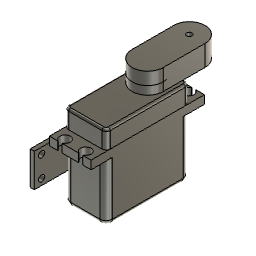
Servo v3 (Autodesk Fusion 360 design; units mm, degrees)
Autodesk Fusion 360 part; units mm, degrees
note: some values were not read from the file. Set by a fixed rule: which sketch regions a step uses.
sketch "Sketch1" plane through (0, 0, 0) normal (0, 0, 1) x (1, 0, 0)
  line L0 (0, 0) -> (20, 0)
  line L1 (20, 0) -> (20, 40)
  line L2 (20, 40) -> (0, 40)
  line L3 (0, 40) -> (0, 0)
  dimension "d1" = 20
  dimension "d2" = 40
  constraint horizontal L0
  constraint vertical L1
  constraint horizontal L2
  constraint vertical L3
  constraint coincident L0.start L3.end
  measures "d1" distance of L1.end L2.end
  measures "d2" distance of L0.end L1.end
extrude "Extrude1" add sketch "Sketch1" along normal blind 27.7 makes body 1
sketch "Sketch2" plane through (0, 0, 27.7) normal (0, 0, 1) x (-1, 0, 0)
  line L0 (0, -40) -> (0, 0)
  line L1 (0, 0) -> (-20, 0)
  line L2 (-20, 0) -> (-20, -40)
  line L3 (-20, -40) -> (0, -40)
  line L4 (0, -47.25) -> (-20, -47.25)
  line L5 (-20, -47.25) -> (-20, 7.25)
  line L6 (-20, 7.25) -> (0, 7.25)
  line L7 (0, 7.25) -> (0, -47.25)
  circle A0 centre (-5, -44.75) radius 2.5
  circle A1 centre (-15, -44.75) radius 2.5
  circle A2 centre (-15, 4.75) radius 2.5
  circle A3 centre (-5, 4.75) radius 2.5
  line L8 (-10, -47.25) -> (-10, 7.25)
  line L9 (-4, -47.25) -> (-6, -47.25)
  line L10 (-6, -47.25) -> (-6, -46.3307)
  line L11 (-6, -46.3307) -> (-4, -46.3307)
  line L12 (-4, -46.3307) -> (-4, -47.25)
  line L13 (-14, -47.25) -> (-16, -47.25)
  line L14 (-16, -47.25) -> (-16, -46.3307)
  line L15 (-16, -46.3307) -> (-14, -46.3307)
  line L16 (-14, -46.3307) -> (-14, -47.25)
  line L17 (-14, 6.8523) -> (-16, 6.8523)
  line L18 (-16, 6.8523) -> (-16, 7.25)
  line L19 (-16, 7.25) -> (-14, 7.25)
  line L20 (-14, 7.25) -> (-14, 6.8523)
  line L21 (-4, 6.8576) -> (-6, 6.8576)
  line L22 (-6, 6.8576) -> (-6, 7.25)
  line L23 (-6, 7.25) -> (-4, 7.25)
  line L24 (-4, 7.25) -> (-4, 6.8576)
  dimension "d5" = 54.5
  dimension "d6" = 20
  dimension "d7" = 10
  dimension "d8" = 10
  dimension "d9" = 10
  dimension "d10" = 5
  dimension "d11" = 5
  dimension "d12" = 2.5
  dimension "d13" = 2.5
  dimension "d14" = 2.5
  dimension "d15" = 2.5
  dimension "d16" = 2
  dimension "d17" = 2
  dimension "d18" = 1
  dimension "d19" = 1
  dimension "d20" = 2
  dimension "d21" = 1
  dimension "d22" = 2
  dimension "d23" = 1
  dimension "d28" = 7.25
  constraint horizontal L4
  constraint vertical L5
  constraint horizontal L6
  constraint vertical L7
  constraint midpoint L4 L8.start
  constraint midpoint L6 L8.end
  constraint tangent L4 A0
  constraint tangent L4 A1
  constraint tangent L6 A3
  constraint tangent L6 A2
  constraint horizontal L9
  constraint vertical L10
  constraint horizontal L11
  constraint vertical L12
  constraint coincident L4 L9.start
  constraint horizontal L13
  constraint vertical L14
  constraint horizontal L15
  constraint vertical L16
  constraint coincident L4 L13.start
  constraint horizontal L17
  constraint vertical L18
  constraint horizontal L19
  constraint vertical L20
  constraint coincident L6 L18.end
  constraint horizontal L21
  constraint vertical L22
  constraint horizontal L23
  constraint vertical L24
  constraint coincident L6 L22.end
  constraint collinear L0 L7
  measures "d5" distance of L4 L6
  measures "d6" distance of L5 L7
  measures "d7" distance of A0.centre A1.centre
  measures "d8" distance of A2.centre A3.centre
  measures "d9" distance of L5 L8
  measures "d10" distance of A1.centre L8
  measures "d11" distance of A2.centre L8
  measures "d12" distance of L6 A3.centre
  measures "d13" distance of L4 A0.centre
  measures "d14" distance of L4 A1.centre
  measures "d15" distance of L6 A2.centre
  measures "d16" distance of L10.end L11.end
  measures "d17" distance of L14.end L15.end
  measures "d18" distance of A1.centre L16
  measures "d19" distance of A0.centre L12
  measures "d20" distance of L21.start L21.end
  measures "d21" distance of A3.centre L24
  measures "d22" distance of L17.start L17.end
  measures "d23" distance of A2.centre L20
  measures "d28" distance of L1 L6
extrude "Extrude2" add sketch "Sketch2" along normal blind 4 contours L0 L1 L3 L7 L8 | L3 L4 L7 A0 L8 L10 L12 | L1 L6 L7 A3 L8 L22 L24 | L3 L4 L5 A1 L8 L14 L16 | L1 L2 L3 L5 L8 | L1 L5 L6 A2 L8 L18 L20 bodies 1
sketch "Sketch3" plane through (0, 0, 31.7) normal (0, 0, 1) x (-1, 0, 0)
  line L0 (0, 7.25) -> (-4, 7.25)
  line L1 (-16, 7.25) -> (-20, 7.25)
  line L2 (-20, 7.25) -> (-20, -47.25)
  line L3 (-20, -47.25) -> (-16, -47.25)
  line L4 (-16, -47.25) -> (-16, -47.0413)
  arc A0 (-14, -47.0413) -> (-16, -47.0413) centre (-15, -44.75) ccw
  line L5 (-14, -47.0413) -> (-14, -47.25)
  line L6 (-14, -47.25) -> (-6, -47.25)
  line L7 (-6, -47.25) -> (-6, -47.0413)
  arc A1 (-4, -47.0413) -> (-6, -47.0413) centre (-5, -44.75) ccw
  line L8 (-4, -47.0413) -> (-4, -47.25)
  line L9 (-4, -47.25) -> (0, -47.25)
  line L10 (0, -47.25) -> (0, 7.25)
  line L11 (0, -40) -> (-20, -40)
  line L12 (-20, -40) -> (-20, 0)
  line L13 (-20, 0) -> (0, 0)
  line L14 (0, 0) -> (0, -40)
  line L15 (-4, 7.25) -> (-4, 7.0413)
  arc A2 (-6, 7.0413) -> (-4, 7.0413) centre (-5, 4.75) ccw
  line L16 (-6, 7.0413) -> (-6, 7.25)
  line L17 (-6, 7.25) -> (-14, 7.25)
  line L18 (-14, 7.25) -> (-14, 7.0413)
  arc A3 (-16, 7.0413) -> (-14, 7.0413) centre (-15, 4.75) ccw
  line L19 (-16, 7.0413) -> (-16, 7.25)
  dimension "d26" = 40
  dimension "d29" = 7.25
  constraint horizontal L11
  constraint vertical L12
  constraint horizontal L13
  constraint vertical L14
  constraint coincident L2 L12.end
  constraint coincident L10 L11.start
  measures "d26" distance of L11.start L13.end
  measures "d29" distance of L0 L13
extrude "Extrude3" add sketch "Sketch3" along normal blind 8.7 separate body contours L2 L10 L11 L12 L13 L14 makes body 2
sketch "Sketch4" plane through (0, 0, 40.4) normal (0, 0, 1) x (-1, 0, 0)
  line L0 (0, 0) -> (-20, 0)
  line L1 (-20, 0) -> (-20, -40)
  line L2 (-20, -40) -> (0, -40)
  line L3 (0, -40) -> (0, 0)
  circle A0 centre (-10, -30) radius 7.5
  line L4 (-2.5, -30) -> (-2.5, -50)
  line L5 (-17.5, -30) -> (-17.5, -50)
  line L6 (-10, -40) -> (-10, 0)
  circle A1 centre (-10, -50) radius 7.5
  circle A2 centre (-10, -50) radius 1.25
  dimension "d32" = 15
  dimension "d33" = 10
  dimension "d44" = 15
  dimension "d45" = 20
  dimension "d46" = 2.5
  constraint coincident A0 L4.start
  constraint parallel L3 L4
  constraint coincident A0 L5.start
  constraint perpendicular L2 L5
  constraint midpoint L2 L6.start
  constraint midpoint L0 L6.end
  constraint coincident A0.centre L6
  constraint tangent A0 L5
  constraint tangent A0 L4
  constraint coincident L5.end A1
  constraint coincident L4.end A1
  constraint tangent L5 A1
  constraint concentric A1 A2
  measures "d32" diameter of A0
  measures "d33" distance of L2 A0.centre
  measures "d44" diameter of A1
  measures "d45" distance of A0.centre A1.centre
  measures "d46" diameter of A2
extrude "Extrude4" add sketch "Sketch4" along normal blind 4 contours A0 L6 | A0 L6 bodies 2
fillet "Fillet1" radius 3 4 edges at (20, 0, 13.85) (0, 0, 13.85) (20, 40, 13.85) (0, 40, 13.85) on bodies 1
fillet "Fillet2" radius 2 8 edges at (0.8787, 0.8787, 0) (10, 0, 0) (19.1213, 0.8787, 0) (20, 20, 0) (19.1213, 39.1213, 0) (10, 40, 0) (0.8787, 39.1213, 0) (0, 20, 0) on bodies 1
fillet "Fillet3" radius 1 4 edges at (0, 20, 40.4) (10, 40, 40.4) (20, 20, 40.4) (10, 0, 40.4) on bodies 2
fillet "Fillet4" radius 2 8 edges at (20, 40, 35.55) (19.7071, 39.7071, 40.1071) (0, 40, 35.55) (0.2929, 39.7071, 40.1071) (0, 0, 35.55) (0.2929, 0.2929, 40.1071) (20, 0, 35.55) (19.7071, 0.2929, 40.1071) on bodies 2
extrude "Extrude5" add sketch "Sketch4" along normal blind 10 separate body contours A0 L6 | A0 L6 | L2 L4 L5 A1 | L2 A0 L4 L6 | L2 A0 L5 L6 | A1 makes body 3
sketch "Sketch5" plane through (0, 0, 0) normal (-1, 0, 0) x (0, -1, 0)
  line L0 (-37, 2) -> (-3, 2)
  line L1 (-3, 2) -> (-3, 27.7)
  line L2 (-3, 27.7) -> (7.25, 27.7)
  line L3 (7.25, 27.7) -> (7.25, 31.7)
  line L4 (7.25, 31.7) -> (-47.25, 31.7)
  line L5 (-47.25, 31.7) -> (-47.25, 27.7)
  line L6 (-47.25, 27.7) -> (-37, 27.7)
  line L7 (-37, 27.7) -> (-37, 2)
  line L8 (-54.5, 29) -> (14.5, 29)
  line L9 (14.5, 29) -> (14.5, 13)
  line L10 (14.5, 13) -> (-54.5, 13)
  line L11 (-54.5, 13) -> (-54.5, 29)
  circle A0 centre (-51, 26) radius 1.5
  circle A1 centre (-51, 16) radius 1.5
  circle A2 centre (11, 26) radius 1.5
  circle A3 centre (11, 16) radius 1.5
  line L12 (-51, 26) -> (11, 26) construction
  line L13 (11, 26) -> (11, 16) construction
  line L14 (11, 16) -> (-51, 16) construction
  line L15 (-51, 16) -> (-51, 26) construction
  line L16 (-54.5, 21) -> (14.5, 21)
  line L17 (11, 21) -> (-51, 21)
  dimension "d49" = 16
  dimension "d50" = 69
  dimension "d51" = 3
  dimension "d52" = 3
  dimension "d53" = 3
  dimension "d54" = 3
  dimension "d55" = 10
  dimension "d56" = 62
  dimension "d57" = 3.5
  dimension "d58" = 69
  dimension "d59" = 69
  dimension "d60" = 11
  dimension "d61" = 17.5
  constraint horizontal L8
  constraint vertical L9
  constraint horizontal L10
  constraint vertical L11
  constraint horizontal L12
  constraint vertical L13
  constraint horizontal L14
  constraint vertical L15
  constraint coincident A3.centre L13.end
  constraint coincident A0.centre L12.start
  constraint coincident A2.centre L12.end
  constraint coincident A1.centre L14.end
  constraint midpoint L11 L16.start
  constraint midpoint L9 L16.end
  constraint midpoint L13 L17.start
  constraint midpoint L15 L17.end
  constraint collinear L16 L17
  measures "d49" distance of L8.start L10.end
  measures "d50" distance of L8.start L8.end
  measures "d51" diameter of A2
  measures "d52" diameter of A3
  measures "d53" diameter of A1
  measures "d54" diameter of A0
  measures "d55" distance of A0.centre A1.centre
  measures "d56" distance of L17.start L17.end
  measures "d57" distance of L11 L15
  measures "d58" distance of L9.end L10.end
  measures "d59" distance of L9.end L10.end
  measures "d60" distance of L0 L10
  measures "d61" distance of L1 L9
extrude "Extrude6" add sketch "Sketch5" along normal blind 2 contours L7 L10 L11 L16 L17 | L1 L7 L10 L16 L17 | L1 L9 L10 L16 L17 | L5 L6 L7 L8 L11 L16 L17 | L1 L2 L3 L5 L6 L7 L8 L16 L17 | L1 L2 L3 L8 L9 L16 L17 bodies 1
